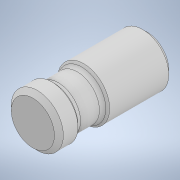
# Autodesk Inventor part: stopper_inhibitory
Saved by Autodesk Inventor 2020 (Build 240168000, 168)
## iProperties
Created: 2019-05-16
Part Number: stopper_inhibitory
Material: 一般
Document SubType Name: Modeling
Designer: yoichi masuda
Density: 1 g/cm^3
Appearance: 既定
Author: yoichi masuda
Autodesk Inventor part; units mm, degrees
ref_plane "YZ Plane" through (0, 0, 0) normal (1, 0, 0) x (0, 1, 0)
ref_plane "XZ Plane" through (0, 0, 0) normal (0, 1, 0) x (-1, 0, 0)
ref_plane "XY Plane" through (0, 0, 0) normal (0, 0, 1) x (1, 0, 0)
sketch "スケッチ1" plane through (0, 0, 0) normal (0, 0, 1) x (1, 0, 0)
  circle A0 centre (0, 0) radius 4.1
  dimension "d0" = 8.2
  constraints: 1 centre point, 1 coincident
  measures "d0" diameter of A0
extrude "押し出し1" add sketch "スケッチ1" along normal blind 10
sketch "スケッチ2" plane through (0, 0, 10) normal (0, 0, 1) x (1, 0, 0)
  circle A0 centre (0, 0) radius 3.5
  dimension "d3" = 7
  constraints: 1 centre point, 1 coincident
  measures "d3" diameter of A0
extrude "押し出し2" add sketch "スケッチ2" along normal blind 5
sketch "スケッチ3" plane through (0, 0, 15) normal (0, 0, 1) x (1, 0, 0)
  circle A0 centre (0, 0) radius 4.1
  circle A1 centre (0, 0) radius 4.1 projected
  circle A2 centre (0, 0) radius 4.1 projected
  point P0 (0, 4.1)
  constraints: 2 vertical alignment, 1 coincident, 3 other
extrude "押し出し3" add sketch "スケッチ3" along normal blind 3
chamfer "面取り1" distance 0.6 angle 45 2 edges at (-3.5, 0, 10) (-3.5, 0, 15)
chamfer "面取り2" distance 0.7 angle 45 2 edges at (-4.1, 0, 18) (-4.1, 0, 0)
fillet "フィレット1" radius 1 2 edges at (-3.5, 0, 10.5995) (-3.5, 0, 14.4005)
